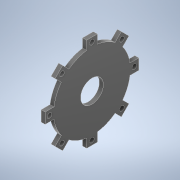
# Autodesk Inventor part: Gear_Box_Chasis_Divider
Saved by Autodesk Inventor 2022 (Build 260153000, 153)
## iProperties
Created: 2022-04-22
Part Number: Gear_Box_Chasis_Divider
Material: ABS Plastic
Document SubType Name: Modeling
Designer: Mlees
Density: 1.06 g/cm^3
Appearance: Smooth - Black
Author: Mlees
Autodesk Inventor part; units mm, degrees
ref_plane "YZ Plane" through (0, 0, 0) normal (1, 0, 0) x (0, 1, 0)
ref_plane "XZ Plane" through (0, 0, 0) normal (0, 1, 0) x (-1, 0, 0)
ref_plane "XY Plane" through (0, 0, 0) normal (0, 0, 1) x (1, 0, 0)
sketch "Sketch1" plane through (0, 0, 0) normal (1, 0, 0) x (0, 1, 0)
  circle A0 centre (0, 0) radius 8.5
  line L0 (28.3441, -4) -> (35, -4)
  line L1 (35, 4) -> (35, -4)
  line L2 (28.3441, 4) -> (35, 4)
  circle A1 centre (31.6721, 0) radius 1.7859
  line L3 (17.2139, 22.8708) -> (21.9203, 27.5772)
  line L4 (21.9203, 27.5772) -> (27.5772, 21.9203)
  circle A2 centre (22.3955, 22.3955) radius 1.7859
  line L5 (22.8708, 17.2139) -> (27.5772, 21.9203)
  line L6 (-4, 28.3441) -> (-4, 35)
  line L7 (-4, 35) -> (4, 35)
  circle A3 centre (0, 31.6721) radius 1.7859
  line L8 (4, 28.3441) -> (4, 35)
  line L9 (-22.8708, 17.2139) -> (-27.5772, 21.9203)
  line L10 (-27.5772, 21.9203) -> (-21.9203, 27.5772)
  circle A4 centre (-22.3955, 22.3955) radius 1.7859
  line L11 (-17.2139, 22.8708) -> (-21.9203, 27.5772)
  line L12 (-28.3441, -4) -> (-35, -4)
  line L13 (-35, -4) -> (-35, 4)
  circle A5 centre (-31.6721, 0) radius 1.7859
  line L14 (-28.3441, 4) -> (-35, 4)
  line L15 (-17.2139, -22.8708) -> (-21.9203, -27.5772)
  line L16 (-21.9203, -27.5772) -> (-27.5772, -21.9203)
  circle A6 centre (-22.3955, -22.3955) radius 1.7859
  line L17 (-22.8708, -17.2139) -> (-27.5772, -21.9203)
  line L18 (4, -28.3441) -> (4, -35)
  line L19 (4, -35) -> (-4, -35)
  circle A7 centre (0, -31.6721) radius 1.7859
  line L20 (-4, -28.3441) -> (-4, -35)
  line L21 (22.8708, -17.2139) -> (27.5772, -21.9203)
  line L22 (27.5772, -21.9203) -> (21.9203, -27.5772)
  circle A8 centre (22.3955, -22.3955) radius 1.7859
  line L23 (17.2139, -22.8708) -> (21.9203, -27.5772)
  arc A9 (22.8708, -17.2139) -> (28.3441, -4) centre (0, 0) ccw
  arc A10 (4, -28.3441) -> (17.2139, -22.8708) centre (0, 0) ccw
  arc A11 (-17.2139, -22.8708) -> (-4, -28.3441) centre (0, 0) ccw
  arc A12 (-28.3441, -4) -> (-22.8708, -17.2139) centre (0, 0) ccw
  arc A13 (-22.8708, 17.2139) -> (-28.3441, 4) centre (0, 0) ccw
  arc A14 (-4, 28.3441) -> (-17.2139, 22.8708) centre (0, 0) ccw
  arc A15 (28.3441, 4) -> (22.8708, 17.2139) centre (0, 0) ccw
  arc A16 (17.2139, 22.8708) -> (4, 28.3441) centre (0, 0) ccw
  dimension "d0" = 17
  dimension "d8" = 360
  constraints: 48 end point, 17 centre point, 16 point on circle, 2 coincident, 1 vertical, 73 other
  measures "d0" diameter of A0
extrude "Extrusion1" add sketch "Sketch1" along normal blind 3
body "Solid1"
